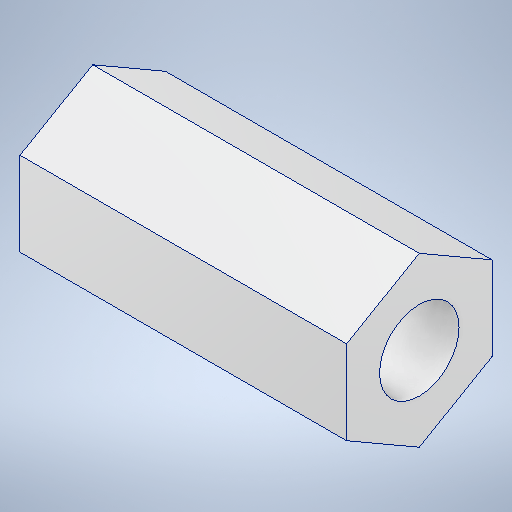
# Autodesk Inventor part: 1.123 hex shaft 0.25-20 0.5
Saved by Autodesk Inventor 2025.1 (Build 291241020, 241B)
## iProperties
Created: 2024-09-18
Part Number: 1.123 hex shaft 0.25-20 0.5
Material: Aluminum 6061
Document SubType Name: Modeling
Designer: xmand
Density: 2.7 g/cm^3
Appearance: Aluminum - Flat
Author: xmand
Autodesk Inventor part; units mm, degrees
ref_plane "YZ Plane" through (0, 0, 0) normal (1, 0, 0) x (0, 1, 0)
ref_plane "XZ Plane" through (0, 0, 0) normal (0, 1, 0) x (-1, 0, 0)
ref_plane "XY Plane" through (0, 0, 0) normal (0, 0, 1) x (1, 0, 0)
sketch "Sketch1" plane through (0, 0, 0) normal (1, 0, 0) x (0, 1, 0)
  circle A0 centre (0, 0) radius 3.4701
  line L0 (7.3323, 0) -> (3.6662, -6.35)
  line L1 (3.6662, -6.35) -> (-3.6662, -6.35)
  line L2 (-3.6662, -6.35) -> (-7.3323, 0)
  line L3 (-7.3323, 0) -> (-3.6662, 6.35)
  line L4 (-3.6662, 6.35) -> (3.6662, 6.35)
  line L5 (3.6662, 6.35) -> (7.3323, 0)
  point P0 (0, -6.35)
  dimension "d0" = 6.9401
  dimension "d1" = 12.7
  constraints: 12 end point, 3 coincident, 1 centre point, 1 horizontal, 1 midpoint, 13 other
  measures "d0" diameter of A0
  measures "d1" distance from line of point (0, -6.35) L4
extrude "Extrusion1" add sketch "Sketch1" along normal mid plane 28.5242
body "Solid1"
